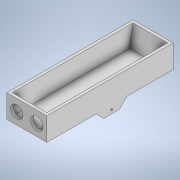
# Autodesk Inventor part: Część1
Saved by Autodesk Inventor 2022.2 (Build 262287010, 287A)
## iProperties
Created: 2023-01-18
Part Number: Część1
Material: Ogólny
Document SubType Name: Modeling
Designer: Miki
Density: 1 g/cm^3
Appearance: Domyślna
Author: Miki
Autodesk Inventor part; units mm, degrees
ref_plane "YZ Plane" through (0, 0, 0) normal (1, 0, 0) x (0, 1, 0)
ref_plane "XZ Plane" through (0, 0, 0) normal (0, 1, 0) x (-1, 0, 0)
ref_plane "XY Plane" through (0, 0, 0) normal (0, 0, 1) x (1, 0, 0)
sketch "Szkic1" plane through (0, 0, 0) normal (0, 1, 0) x (-1, 0, 0)
  line L0 (-26, 80) -> (26, 80)
  line L1 (26, 80) -> (26, -80)
  line L2 (26, -80) -> (-26, -80)
  line L3 (-26, -80) -> (-26, 80)
  line L4 (-26, 80) -> (26, -80) construction
  line L5 (26, 80) -> (-26, -80) construction
  point P0 (0, 0)
  dimension "d0" = 52
  dimension "d1" = 160
  constraints: 12 end point, 2 midpoint, 2 parallel, 1 horizontal, 1 perpendicular
  measures "d0" distance of L1.end L2.end
  measures "d1" distance of L0.end L1.end
extrude "Wyciągnięcie proste1" add sketch "Szkic1" along normal blind 30
shell "Skorupa1" thickness 3.5 removed faces 1 at (8.6667, 30, 26.6667)
sketch "Szkic3" plane through (-26, 0, 80) normal (0, 0, 1) x (1, 0, 0)
  line L0 (52, 0) -> (52, 30) projected
  line L1 (0, 0) -> (52, 0)
  line L2 (52, 0) -> (52, 30)
  line L3 (52, 30) -> (0, 30)
  line L4 (0, 30) -> (0, 0)
  line L5 (52, 0) -> (0, 0) projected
  line L6 (52, 30) -> (0, 30) projected
  line L7 (48.5, 0) -> (3.5, 0)
  line L8 (3.5, 0) -> (3.5, 30)
  line L9 (3.5, 30) -> (48.5, 30)
  line L10 (48.5, 30) -> (48.5, 0)
  line L11 (3.5, 25) -> (48.5, 25)
  line L12 (48.5, 25) -> (48.5, 5)
  line L13 (48.5, 5) -> (3.5, 5)
  line L14 (3.5, 5) -> (3.5, 25)
  circle A0 centre (13, 15) radius 8
  circle A1 centre (39, 15) radius 8
  point P0 (26, 0)
  point P1 (3.5, 15)
  dimension "d7" = 52
  dimension "d8" = 30
  dimension "d9" = 3.5
  dimension "d10" = 3.5
  dimension "d11" = 45
  dimension "d12" = 45
  dimension "d13" = 20
  dimension "d14" = 5
  dimension "d15" = 16
  dimension "d16" = 16
  dimension "d17" = 26
  dimension "d18" = 10
  dimension "d19" = 9.5
  constraints: 24 end point, 6 parallel, 4 point on line, 3 horizontal, 3 perpendicular, 2 centre point, 1 horizontal alignment, 1 midpoint
  measures "d7" distance of L1.start L1.end
  measures "d8" distance of L0.start L0.end
  measures "d9" distance between parallel lines of L4 L8
  measures "d10" distance between parallel lines of L0 L10
  measures "d11" distance between parallel lines of L10 L8
  measures "d12" distance of L12.end L13.end
  measures "d13" distance between parallel lines of L13 L11
  measures "d14" distance between parallel lines of L3 L11
  measures "d15" diameter of A0
  measures "d16" diameter of A1
  measures "d17" distance of A1.centre A0.centre
  measures "d18" distance from line of L13 A0.centre
  measures "d19" distance of point (3.5, 15) A0.centre
extrude "Wyciągnięcie proste2" cut sketch "Szkic3" against normal up to next contours A0 | A1
sketch "Szkic4" plane through (-26, 0, 80) normal (0, 0, 1) x (1, 0, 0)
  line L0 (0, 0) -> (0, 30) projected
  line L1 (0, 30) -> (52, 30) projected
  line L2 (0, 0) -> (52, 0)
  line L3 (52, 0) -> (52, 30)
  line L4 (52, 30) -> (0, 30)
  line L5 (0, 30) -> (0, 0)
  circle A0 centre (13, 15) radius 8 projected
  circle A1 centre (13, 15) radius 8
  circle A2 centre (39, 15) radius 8 projected
  circle A3 centre (39, 15) radius 8
  point P0 (26, 0)
  point P1 (47, 22.5)
  constraints: 8 end point, 2 centre point, 2 coincident, 2 parallel, 1 horizontal, 1 perpendicular, 1 other
extrude "Wyciągnięcie proste3" add sketch "Szkic4" along normal blind 4
sketch "Szkic8" plane through (0, 0, 0) normal (0, -1, 0) x (1, 0, 0)
  line L0 (26, 10) -> (22, 10)
  line L1 (22, 10) -> (22, -10)
  line L2 (22, -10) -> (26, -10)
  line L3 (26, -10) -> (26, 10)
  line L4 (26, -80) -> (26, 84) projected
  point P0 (0, 0)
  point P1 (26, 0)
  point P2 (26, 2)
  dimension "d46" = 20
  dimension "d47" = 4
  constraints: 8 end point, 2 midpoint, 2 parallel, 1 horizontal, 1 horizontal alignment, 1 perpendicular, 1 vertical alignment
  measures "d46" distance of L2.end L0.start
  measures "d47" distance of L1.end L2.end
extrude "Wyciągnięcie proste6" add sketch "Szkic8" along normal blind 10
sketch "Szkic9" plane through (22, 0, -10) normal (-1, 0, 0) x (0, 0, 1)
  circle A0 centre (10, -5) radius 1.25
  line L0 (0, 0) -> (20, 0) projected
  line L1 (20, 0) -> (20, -10) projected
  point P0 (10, 0)
  point P1 (10, 0)
  point P2 (20, -5)
  dimension "d50" = 2.5
  constraints: 2 midpoint, 1 centre point, 1 horizontal alignment, 1 vertical alignment
  measures "d50" diameter of A0
extrude "Wyciągnięcie proste7" cut sketch "Szkic9" against normal up to next
sketch "Szkic11" plane through (0, 0, 0) normal (0, -1, 0) x (1, 0, 0)
  line L0 (-26, -80) -> (-26, 84) projected
  line L1 (-26, 15) -> (-22, 15)
  line L2 (-22, 15) -> (-22, -15)
  line L3 (-22, -15) -> (-26, -15)
  line L4 (-26, -15) -> (-26, 15)
  point P0 (0, 0)
  dimension "d55" = 4
  dimension "d56" = 30
  dimension "d57" = 15
  constraints: 8 end point, 2 parallel, 1 horizontal, 1 perpendicular, 1 point on line
  measures "d55" distance of L2.end L3.end
  measures "d56" distance of L1.end L2.end
  measures "d57" vertical distance of L1.start point (0, 0)
extrude "Wyciągnięcie proste8" add sketch "Szkic11" along normal blind 20
sketch "Szkic12" plane through (-26, 0, -80) normal (-1, 0, 0) x (0, 0, 1)
  circle A0 centre (80, -10) radius 5
  line L0 (95, 0) -> (95, -20) projected
  line L1 (95, -20) -> (65, -20) projected
  point P0 (80, 0)
  dimension "d60" = 10
  dimension "d61" = 15
  dimension "d62" = 10
  constraints: 1 centre point
  measures "d60" diameter of A0
  measures "d61" distance from line of L0 A0.centre
  measures "d62" distance from line of L1 A0.centre
extrude "Wyciągnięcie proste9" cut sketch "Szkic12" against normal blind 20
sketch "Szkic13" plane through (-26, 0, -80) normal (-1, 0, 0) x (0, 0, 1)
  line L0 (95, -20) -> (65, -20) projected
  line L1 (95, -20) -> (109.2717, -5.7283)
  line L2 (95, -20) -> (115.1833, -20) construction
  line L3 (109.2717, -5.7283) -> (115, 0)
  line L4 (95, 0) -> (164, 0) projected
  line L5 (95, 0) -> (95, -20) projected
  line L6 (95, 0) -> (95, -20)
  line L7 (65, 0) -> (65, -20) projected
  line L8 (65, -20) -> (48.9371, -3.9371)
  line L9 (65, -20) -> (87.7163, -20) construction
  line L10 (48.9371, -3.9371) -> (45, 0)
  line L11 (0, 0) -> (70, 0) projected
  line L12 (95, 0) -> (65, 0) projected
  line L13 (65, 0) -> (65, -20)
  line L14 (65, 0) -> (45, 0)
  line L15 (115, 0) -> (95, 0)
  point P0 (80, 0)
  dimension "d65" = 45
  dimension "d67" = 135
  constraints: 20 end point, 4 point on line, 2 collinear, 2 equal length, 2 horizontal, 2 perpendicular
  measures "d65" angle of L2 L1
  measures "d67" angle of L9 L8
extrude "Wyciągnięcie proste10" add sketch "Szkic13" against normal blind 4 contours L5 L4 L3 L1 | L8 L10 L11 L7
sketch "Szkic14" plane through (26, 0, -80) normal (1, 0, 0) x (0, 0, -1)
  line L0 (-70, -10) -> (-60, 0)
  line L1 (-70, -10) -> (-55.8579, -10) construction
  line L2 (-70, 0) -> (-70, -10) projected
  line L3 (-60, 0) -> (-70, 0)
  line L4 (-70, 0) -> (-70, -10)
  line L5 (-90, 0) -> (-90, -10) projected
  line L6 (-90, -10) -> (-100, 0)
  line L7 (-90, -10) -> (-75.8579, -10) construction
  line L8 (-100, 0) -> (-90, 0)
  line L9 (-90, 0) -> (-90, -10)
  point P0 (-80, 0)
  point P1 (-115, 0)
  point P2 (-45, 0)
  dimension "d70" = 45
  dimension "d71" = 135
  constraints: 16 end point, 3 perpendicular, 2 equal length, 2 horizontal, 1 collinear
  measures "d70" angle of L1 L0
  measures "d71" angle of L7 L6
extrude "Wyciągnięcie proste11" add sketch "Szkic14" against normal blind 4
sketch "Szkic15" plane through (22.5, 3.5, 76.5) normal (0, 0, -1) x (-1, 0, 0)
  line L0 (0, 26.5) -> (45, 26.5) projected
  line L1 (45, 26.5) -> (0, 26.5)
  line L2 (0, 26.5) -> (0, -1)
  line L3 (0, -1) -> (45, -1)
  line L4 (45, -1) -> (45, 26.5)
  point P0 (22.5, -3.5)
  point P1 (0, 26.5)
  dimension "d74" = 27.5
  constraints: 8 end point, 2 parallel, 1 horizontal, 1 perpendicular
  measures "d74" distance between parallel lines of L0 L3
extrude "Wyciągnięcie proste12" cut sketch "Szkic15" against normal blind 4
sketch "Szkic17" plane through (-22.5, 3.5, -76.5) normal (1, 0, 0) x (0, 0, -1)
  line L0 (0, 26.5) -> (-4.1115, 3.1827)
  line L1 (0, 26.5) -> (23.677, 26.5) construction
  line L2 (-4.1115, 3.1827) -> (-5.1108, -2.485)
  line L3 (-4.6727, 0) -> (0, 0)
  line L4 (-157, 26.5) -> (0, 26.5) projected
  line L5 (0, 0) -> (0, 26.5)
  point P0 (-76.5, -3.5)
  dimension "d77" = 100
  constraints: 10 end point, 2 horizontal, 2 point on line, 1 equal length, 1 perpendicular
  measures "d77" angle of L0 L1
extrude "Wyciągnięcie proste13" add sketch "Szkic17" along normal blind 48
sketch "Szkic20" plane through (22.5, 3.5, 76.5) normal (0, 0, 1) x (1, 0, 0)
  line L0 (0, -1) -> (0, 26.5) projected
  line L1 (-45, 0) -> (0, 0)
  line L2 (0, 0) -> (0, -1)
  line L3 (0, -1) -> (-45, -1)
  line L4 (-45, -1) -> (-45, 0)
  point P0 (-22.5, -3.5)
  constraints: 8 end point, 2 parallel, 1 horizontal, 1 perpendicular
extrude "Wyciągnięcie proste14" add sketch "Szkic20" along normal blind 7
equation "\"d10\" = d9"
equation "\"d14\" = -0.5 * d13 + 0.5 * d8"
equation "\"d18\" = 0.5 * d13"
